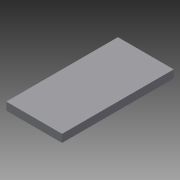
# Autodesk Inventor part: Level1
Saved by Autodesk Inventor 2015 (Build 190159000, 159)
## iProperties
Created: 2015-08-18
Part Number: Level1
Material: Generic
Document SubType Name: Modeling
Designer: pkurlak
Density: 1 g/cm^3
Appearance: Default
Author: pkurlak
Autodesk Inventor part; units mm, degrees
ref_plane "YZ Plane" through (0, 0, 0) normal (1, 0, 0) x (0, 1, 0)
ref_plane "XZ Plane" through (0, 0, 0) normal (0, 1, 0) x (-1, 0, 0)
ref_plane "XY Plane" through (0, 0, 0) normal (0, 0, 1) x (1, 0, 0)
sketch "Sketch1" plane through (0, 0, 0) normal (0, 1, 0) x (-1, 0, 0)
  line L0 (12736.5103, 30135.77) -> (-17743.4897, 30135.77)
  line L1 (-17743.4897, 30135.77) -> (-17743.4897, -30824.23)
  line L2 (-17743.4897, -30824.23) -> (12736.5103, -30824.23)
  line L3 (12736.5103, -30824.23) -> (12736.5103, 30135.77)
  line L4 (11554.7803, 29000.7039) -> (8879.6143, 29000.7039)
  line L5 (8879.6143, 29000.7039) -> (8879.6143, -26249.6646)
  line L6 (11554.7803, -29579.9734) -> (11554.7803, 29000.7039)
  line L7 (8879.6143, -26249.6646) -> (5603.9009, -26249.6646)
  line L8 (-2503.4897, -1954.7891) -> (-2503.4897, -29579.9734)
  line L9 (-2503.4897, -26249.6646) -> (-2503.4897, -1954.7891)
  line L10 (5603.9009, -1954.7891) -> (5603.9009, -26249.6646)
  line L11 (3188.0623, -1954.7891) -> (3188.0623, 14041.612)
  line L12 (5003.3535, 11038.8746) -> (5003.3535, -1954.7891)
  line L13 (-1875.6447, -1954.7891) -> (-1875.6447, 11038.8746)
  line L14 (-1875.6447, 11038.8746) -> (-1384.2877, 11038.8746)
  line L15 (417.3547, 14041.612) -> (417.3547, -1954.7891)
  line L16 (-7225.9766, 6452.8756) -> (-7225.9766, 14041.612)
  line L17 (-7225.9766, 14041.612) -> (417.3547, 14041.612)
  line L18 (417.3547, 14041.612) -> (417.3547, -1954.7891)
  line L19 (-4605.4058, 11038.8746) -> (-5424.3342, 11038.8746)
  line L20 (5003.3535, 11038.8746) -> (7896.9003, 11038.8746)
  line L21 (7896.9003, 11038.8746) -> (7896.9003, 14041.612)
  line L22 (5603.9009, 14041.612) -> (3188.0623, 14041.612)
  line L23 (3188.0623, 14041.612) -> (3188.0623, 11038.8746)
  line L24 (5603.9009, 14041.612) -> (5603.9009, 19610.3251)
  line L25 (5603.9009, 27308.2519) -> (7896.9003, 27308.2519)
  line L26 (7896.9003, 27308.2519) -> (7896.9003, 11038.8746)
  line L27 (7896.9003, 27308.2519) -> (-7771.9288, 27308.2519)
  line L28 (-7771.9288, 27308.2519) -> (-7771.9288, 22176.3007)
  line L29 (-9355.1903, 19610.3251) -> (5603.9009, 19610.3251)
  line L30 (-13067.6654, 22176.3007) -> (-13067.6654, 19610.3251)
  line L31 (-13067.6654, 22176.3007) -> (-13067.6654, -21499.88)
  line L32 (-10938.4517, -20298.785) -> (-10938.4517, 19610.3251)
  line L33 (-17216.9024, 7544.7802) -> (-17216.9024, -23356.1177)
  line L34 (-17216.9024, -23356.1177) -> (-4605.4058, -23356.1177)
  line L35 (-4605.4058, -23356.1177) -> (-4605.4058, -20298.785)
  line L36 (-17216.9024, 28727.7278) -> (-14923.903, 28727.7278)
  line L37 (-16507.1645, 7544.7802) -> (-17216.9024, 7544.7802)
  line L38 (-17216.9024, 8800.4703) -> (-16507.1645, 8800.4703)
  line L39 (-16507.1645, 8800.4703) -> (-16507.1645, 7544.7802)
  line L40 (-14923.903, 18300.0396) -> (-16070.4027, 18300.0396)
  line L41 (-16070.4027, 18300.0396) -> (-16070.4027, 20674.932)
  line L42 (-16070.4027, 20674.932) -> (-14923.903, 20674.932)
  line L43 (-14923.903, 18300.0396) -> (-14923.903, -21499.88)
  line L44 (-14923.903, -21499.88) -> (-13067.6654, -21499.88)
  line L45 (-13067.6654, -21499.88) -> (-13067.6654, 22176.3007)
  line L46 (-7225.9766, 3941.4952) -> (-6570.8339, 3941.4952)
  line L47 (-6570.8339, 3941.4952) -> (-6570.8339, 6452.8756)
  line L48 (-6570.8339, 6452.8756) -> (-7225.9766, 6452.8756)
  line L49 (-4605.4058, 2522.0194) -> (-5424.3342, 2522.0194)
  line L50 (-5424.3342, 2522.0194) -> (-5424.3342, -344.23)
  line L51 (-5424.3342, -344.23) -> (-4605.4058, -344.23)
  line L52 (-7225.9766, -1954.7891) -> (-6243.2625, -1954.7891)
  line L53 (-6243.2625, -1954.7891) -> (-6243.2625, -4629.9552)
  line L54 (-6243.2625, -4629.9552) -> (-7225.9766, -4629.9552)
  line L55 (-4605.4058, -5831.0502) -> (-5424.3342, -5831.0502)
  line L56 (-5424.3342, -5831.0502) -> (-5424.3342, -8670.0019)
  line L57 (-5424.3342, -8670.0019) -> (-4605.4058, -8670.0019)
  line L58 (-7225.9766, -10253.2635) -> (-6243.2625, -10253.2635)
  line L59 (-6243.2625, -10253.2635) -> (-6243.2625, -12710.0486)
  line L60 (-6243.2625, -12710.0486) -> (-7225.9766, -12710.0486)
  line L61 (-4605.4058, -14620.8815) -> (-5915.6912, -14620.8815)
  line L62 (-5915.6912, -14620.8815) -> (-5915.6912, -16750.0953)
  line L63 (-5915.6912, -16750.0953) -> (-4605.4058, -16750.0953)
  line L64 (-1384.2877, 11038.8746) -> (-1384.2877, 11857.803)
  line L65 (-1384.2877, 11857.803) -> (-5424.3342, 11857.803)
  line L66 (-5424.3342, 11857.803) -> (-5424.3342, 11038.8746)
  line L67 (-7225.9766, -20298.785) -> (-10938.4517, -20298.785)
  line L68 (-17216.9024, -20298.785) -> (-17216.9024, 7544.7802)
  line L69 (-17216.9024, 8800.4703) -> (-17216.9024, 28727.7278)
  line L70 (-14923.903, 28727.7278) -> (-14923.903, 20674.932)
  line L71 (-14923.903, 18300.0396) -> (-14923.903, -21499.88)
  line L72 (5003.3535, -1954.7891) -> (5603.9009, -1954.7891)
  line L73 (-2503.4897, -1954.7891) -> (-1875.6447, -1954.7891)
  line L74 (417.3547, -1954.7891) -> (3188.0623, -1954.7891)
  line L75 (-1384.2877, 11038.8746) -> (-1875.6447, 11038.8746)
  line L76 (-4605.4058, 11038.8746) -> (-5424.3342, 11038.8746)
  line L77 (-5424.3342, 11038.8746) -> (-4605.4058, 11038.8746)
  line L78 (-1875.6447, 11038.8746) -> (-1384.2877, 11038.8746)
  line L79 (-7225.9766, 11038.8746) -> (-7225.9766, 6452.8756)
  line L80 (-7225.9766, 3941.4952) -> (-7225.9766, -1954.7891)
  line L81 (-4605.4058, 2522.0194) -> (-4605.4058, 11038.8746)
  line L82 (-4605.4058, -5831.0502) -> (-4605.4058, -344.23)
  line L83 (-4605.4058, -23356.1177) -> (-4605.4058, -16750.0953)
  line L84 (-4605.4058, -14620.8815) -> (-4605.4058, -8670.0019)
  line L85 (-7225.9766, -4629.9552) -> (-7225.9766, -10253.2635)
  line L86 (-7225.9766, -12710.0486) -> (-7225.9766, -20298.785)
  line L87 (-10419.7971, 19610.3251) -> (-10419.7971, 22176.3007)
  line L88 (-9355.1903, 22176.3007) -> (-9355.1903, 19610.3251)
  line L89 (-10938.4517, 19610.3251) -> (-10419.7971, 19610.3251)
  line L90 (-9355.1903, 19610.3251) -> (-7771.9288, 19610.3251)
  line L91 (-7771.9288, 22176.3007) -> (-9355.1903, 22176.3007)
  line L92 (-10419.7971, 22176.3007) -> (-13067.6654, 22176.3007)
  line L93 (11554.7803, -29579.9734) -> (-2503.4897, -29579.9734)
  point P0 (0, 0)
  dimension "d0" = 60960
  dimension "d1" = 30480
  dimension "d2" = 2675.1659
  constraints: 188 end point, 53 parallel, 25 perpendicular, 21 horizontal, 11 point on line
  measures "d0" distance of L0.end L1.end
  measures "d1" distance of L1.end L2.end
  measures "d2" distance of L4.start L4.end
extrude "Extrusion1" add sketch "Sketch1" along normal blind 3657.6
sketch "Sketch2" plane through (0, 0, 0) normal (0, -1, 0) x (1, 0, 0)
  line L0 (17743.4897, 30135.77) -> (-12736.5103, 30135.77)
  line L1 (-12736.5103, 30135.77) -> (-12736.5103, -30824.23)
  line L2 (-12736.5103, -30824.23) -> (17743.4897, -30824.23)
  line L3 (17743.4897, -30824.23) -> (17743.4897, 30135.77)
  point P0 (0, 0)
  constraints: 8 end point, 2 parallel, 1 horizontal, 1 perpendicular
extrude "Extrusion2" add sketch "Sketch2" along normal blind 304.8
sketch "Sketch3" plane through (0, 3657.6, 0) normal (0, 1, 0) x (1, 0, 0)
  line L0 (-12736.5103, 30824.23) -> (17743.4897, 30824.23)
  line L1 (17743.4897, 30824.23) -> (17743.4897, -30135.77)
  line L2 (17743.4897, -30135.77) -> (-12736.5103, -30135.77)
  line L3 (-12736.5103, -30135.77) -> (-12736.5103, 30824.23)
  point P0 (0, 0)
  constraints: 8 end point, 2 parallel, 1 horizontal, 1 perpendicular
extrude "Extrusion3" add sketch "Sketch3" along normal blind 304.8
body "Solid1"
